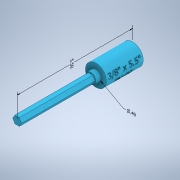
# Autodesk Inventor part: 3_8x7_5-inchHexShaft
Saved by Autodesk Inventor 2022.2 (Build 262287030, 287C)
## iProperties
Created: 2020-11-17
Part Number: 3_8x7_5-inchHexShaft
Material: PC/ABS Plastic
Document SubType Name: Modeling
Designer: robst
Density: 0.357273 g/cm^3
Appearance: Turquoise
Author: robst
Autodesk Inventor part; units mm, degrees
ref_plane "XZ Plane" through (0, 0, 0) normal (0, 1, 0) x (-1, 0, 0)
ref_plane "XY Plane" through (0, 0, 0) normal (0, 0, 1) x (1, 0, 0)
sketch "Sketch1" plane through (0, 0, 0) normal (0, 0, 1) x (1, 0, 0)
  line L0 (5.4993, 0) -> (2.7496, -4.7625)
  line L1 (2.7496, -4.7625) -> (-2.7496, -4.7625)
  line L2 (-2.7496, -4.7625) -> (-5.4993, 0)
  line L3 (-5.4993, 0) -> (-2.7496, 4.7625)
  line L4 (-2.7496, 4.7625) -> (2.7496, 4.7625)
  line L5 (2.7496, 4.7625) -> (5.4993, 0)
  circle A0 centre (0, 0) radius 0.0127
  dimension "d0" = 9.525
  dimension "d6" = 0.0254
  constraints: 12 end point, 2 coincident, 1 centre point, 1 horizontal, 13 other
  measures "d0" distance between parallel lines of L1 L4
  measures "d6" diameter of A0
extrude "Extrusion2" add sketch "Sketch1" along normal mid plane 114.3
sketch "Sketch4" plane through (0, 0, -57.15) normal (0, 0, -1) x (-1, 0, 0)
  circle A0 centre (0, 0) radius 0.0127 projected
  circle A1 centre (0, 0) radius 12.7
  dimension "d10" = 25.4
  constraints: 1 centre point, 1 coincident
  measures "d10" diameter of A1
extrude "Extrusion4" add sketch "Sketch4" against normal blind 19.05
thicken "Reduce Hex Shaft" operation add thickness 0.127 both sides no extend neighbours yes toward (0, -1, 0) faces at (0.9165, 4.7625, -6.35) (4.5827, 1.5875, -6.35) (3.6662, -3.175, -6.35) (-3.6662, 3.175, -6.35) (-4.5827, -1.5875, -6.35) (-0.9165, -4.7625, -6.35)
sketch "Sketch5" plane through (0, 0, -38.1) normal (0, 0, 1) x (1, 0, 0)
  circle A0 centre (0, 0) radius 6.35
  dimension "d15" = 12.7
  constraints: 1 centre point, 1 coincident
  measures "d15" diameter of A0
extrude "Extrusion5" add sketch "Sketch5" along normal blind 6.35
thicken "Reduce Base Bushing" operation add thickness 0.127 both sides no extend neighbours yes toward (-0.9967573, 0.0804666, 0) faces at (6.3294, -0.511, -33.8667)
sketch "Sketch8" plane through (0, 0, -57.15) normal (0, 0, -1) x (-1, 0, 0)
  circle A0 centre (0, 0) radius 12.7
  circle A1 centre (0, 0) radius 12.7 projected
  constraints: 1 centre point, 1 coincident, 1 concentric
extrude "Extrusion7" add sketch "Sketch8" along normal blind 25.4
ref_plane "Work Plane1" through (12.7, 0, -57.15) normal (1, 0, 0) x (0, 1, 0)
sketch "Sketch10" plane through (12.7, 0, -57.15) normal (1, 0, 0) x (0, 1, 0)
  line L0 (-12.7, -25.4) -> (12.7, -25.4) projected
  line L1 (12.7, 19.05) -> (-12.7, 19.05) projected
  line L2 (-6.223, 19.05) -> (6.223, 19.05) construction
  line L3 (0, 19.05) -> (0, -25.4) construction
  spline S0 degree 2 poles (5.518, 14.8141) (5.518, 15.0364) (5.4093, 15.4761) (5.3254, 15.6885) knots 0 0 0 1 2 2 2
  spline S1 degree 2 poles (5.3254, 15.6885) (5.2414, 15.8861) (5.0635, 16.1776) (4.9845, 16.2912) knots 0 0 0 1 2 2 2
  line L4 (4.9845, 16.2912) -> (4.9845, 16.3406)
  line L5 (4.9845, 16.3406) -> (5.849, 16.3406)
  spline S2 degree 2 poles (5.849, 16.3406) (5.9923, 16.0738) (6.2244, 15.1599) (6.2244, 14.7499) knots 0 0 0 1 2 2 2
  spline S3 degree 2 poles (6.2244, 14.7499) (6.2244, 14.3349) (6.0565, 13.7174) (5.8786, 13.4655) knots 0 0 0 1 2 2 2
  spline S4 degree 2 poles (5.8786, 13.4655) (5.686, 13.1987) (5.1278, 12.9221) (4.7523, 12.9221) knots 0 0 0 1 2 2 2
  spline S5 degree 2 poles (4.7523, 12.9221) (4.2484, 12.9221) (3.4877, 13.5841) (3.3889, 14.0484) knots 0 0 0 1 2 2 2
  line L6 (3.3889, 14.0484) -> (3.3296, 14.0484)
  spline S6 degree 2 poles (3.3296, 14.0484) (3.2901, 13.8558) (3.1122, 13.4161) (2.9344, 13.2284) knots 0 0 0 1 2 2 2
  spline S7 degree 2 poles (2.9344, 13.2284) (2.7615, 13.0407) (2.2082, 12.8035) (1.8081, 12.8035) knots 0 0 0 1 2 2 2
  spline S8 degree 2 poles (1.8081, 12.8035) (1.398, 12.8035) (0.7015, 13.0851) (0.4347, 13.342) knots 0 0 0 1 2 2 2
  spline S9 degree 2 poles (0.4347, 13.342) (0.1581, 13.6088) (-0.1284, 14.3646) (-0.1284, 14.8438) knots 0 0 0 1 2 2 2
  spline S10 degree 2 poles (-0.1284, 14.8438) (-0.1284, 15.3032) (0.0939, 16.2023) (0.247, 16.5086) knots 0 0 0 1 2 2 2
  line L7 (0.247, 16.5086) -> (1.1115, 16.5086)
  line L8 (1.1115, 16.5086) -> (1.1115, 16.4493)
  spline S11 degree 2 poles (1.1115, 16.4493) (0.9238, 16.1924) (0.578, 15.323) (0.578, 14.8932) knots 0 0 0 1 2 2 2
  spline S12 degree 2 poles (0.578, 14.8932) (0.578, 14.6412) (0.7361, 14.1373) (0.9188, 13.9694) knots 0 0 0 1 2 2 2
  spline S13 degree 2 poles (0.9188, 13.9694) (1.1016, 13.8064) (1.5364, 13.6335) (1.8673, 13.6335) knots 0 0 0 1 2 2 2
  spline S14 degree 2 poles (1.8673, 13.6335) (2.1983, 13.6335) (2.6281, 13.8261) (2.7516, 13.999) knots 0 0 0 1 2 2 2
  spline S15 degree 2 poles (2.7516, 13.999) (2.8751, 14.1719) (2.969, 14.6412) (2.969, 14.9179) knots 0 0 0 1 2 2 2
  line L9 (2.969, 14.9179) -> (2.969, 15.2637)
  line L10 (2.969, 15.2637) -> (3.6457, 15.2637)
  line L11 (3.6457, 15.2637) -> (3.6457, 14.992)
  spline S16 degree 2 poles (3.6457, 14.992) (3.6457, 14.4436) (4.1694, 13.752) (4.6683, 13.752) knots 0 0 0 1 2 2 2
  spline S17 degree 2 poles (4.6683, 13.752) (4.9005, 13.752) (5.2315, 13.9299) (5.3303, 14.0731) knots 0 0 0 1 2 2 2
  spline S18 degree 2 poles (5.3303, 14.0731) (5.434, 14.2263) (5.518, 14.6017) (5.518, 14.8141) knots 0 0 0 1 2 2 2
  line L12 (6.3677, 9.3505) -> (-1.3239, 11.7365)
  line L13 (-1.3239, 11.7365) -> (-1.3239, 12.4281)
  line L14 (-1.3239, 12.4281) -> (6.3677, 10.0519)
  line L15 (6.3677, 10.0519) -> (6.3677, 9.3505)
  spline S19 degree 2 poles (-0.1383, 6.836) (-0.1383, 7.2905) (0.1334, 8.0364) (0.3853, 8.2982) knots 0 0 0 1 2 2 2
  spline S20 degree 2 poles (0.3853, 8.2982) (0.6323, 8.5551) (1.3042, 8.8219) (1.6846, 8.8219) knots 0 0 0 1 2 2 2
  spline S21 degree 2 poles (1.6846, 8.8219) (2.1786, 8.8219) (3.0085, 8.2933) (3.2555, 7.7894) knots 0 0 0 1 2 2 2
  line L16 (3.2555, 7.7894) -> (3.2802, 7.7894)
  spline S22 degree 2 poles (3.2802, 7.7894) (3.542, 8.2389) (4.1644, 8.6737) (4.6288, 8.6737) knots 0 0 0 1 2 2 2
  spline S23 degree 2 poles (4.6288, 8.6737) (5.3155, 8.6737) (6.2343, 7.6363) (6.2343, 6.836) knots 0 0 0 1 2 2 2
  spline S24 degree 2 poles (6.2343, 6.836) (6.2343, 6.0061) (5.3649, 5.0032) (4.6832, 5.0032) knots 0 0 0 1 2 2 2
  spline S25 degree 2 poles (4.6832, 5.0032) (4.2731, 5.0032) (3.4728, 5.4824) (3.2456, 5.9319) knots 0 0 0 1 2 2 2
  line L17 (3.2456, 5.9319) -> (3.2209, 5.9319)
  spline S26 degree 2 poles (3.2209, 5.9319) (2.9739, 5.3984) (2.2625, 4.8501) (1.6994, 4.8501) knots 0 0 0 1 2 2 2
  spline S27 degree 2 poles (1.6994, 4.8501) (0.9188, 4.8501) (-0.1383, 5.9863) (-0.1383, 6.836) knots 0 0 0 1 2 2 2
  spline S28 degree 2 poles (1.6203, 5.6899) (1.9958, 5.6899) (2.4404, 5.9863) (2.6676, 6.4062) knots 0 0 0 1 2 2 2
  spline S29 degree 2 poles (2.6676, 6.4062) (2.7467, 6.5445) (2.9294, 7.0089) (3.048, 7.3003) knots 0 0 0 1 2 2 2
  spline S30 degree 2 poles (3.048, 7.3003) (2.8257, 7.6363) (2.1637, 7.9969) (1.7438, 7.9969) knots 0 0 0 1 2 2 2
  spline S31 degree 2 poles (1.7438, 7.9969) (1.1905, 7.9969) (0.4693, 7.33) (0.4693, 6.8261) knots 0 0 0 1 2 2 2
  spline S32 degree 2 poles (0.4693, 6.8261) (0.4693, 6.3123) (1.0868, 5.6899) (1.6203, 5.6899) knots 0 0 0 1 2 2 2
  spline S33 degree 2 poles (4.6733, 5.8035) (5.0833, 5.8035) (5.6316, 6.3519) (5.6316, 6.8409) knots 0 0 0 1 2 2 2
  spline S34 degree 2 poles (5.6316, 6.8409) (5.6316, 7.2855) (5.1426, 7.8536) (4.7227, 7.8536) knots 0 0 0 1 2 2 2
  spline S35 degree 2 poles (4.7227, 7.8536) (4.4213, 7.8536) (4.0014, 7.5622) (3.8335, 7.2707) knots 0 0 0 1 2 2 2
  spline S36 degree 2 poles (3.8335, 7.2707) (3.7643, 7.1472) (3.5222, 6.6236) (3.4531, 6.4111) knots 0 0 0 1 2 2 2
  spline S37 degree 2 poles (3.4531, 6.4111) (3.7248, 6.0555) (4.3028, 5.8035) (4.6733, 5.8035) knots 0 0 0 1 2 2 2
  line L18 (6.3677, 1.6489) -> (3.9965, 1.8268)
  line L19 (3.9965, 1.8268) -> (3.9965, 2.3652)
  line L20 (3.9965, 2.3652) -> (6.3677, 2.5431)
  line L21 (6.3677, 2.5431) -> (6.3677, 1.6489)
  line L22 (6.3677, 3.1902) -> (3.9965, 3.3681)
  line L23 (3.9965, 3.3681) -> (3.9965, 3.9065)
  line L24 (3.9965, 3.9065) -> (6.3677, 4.0844)
  line L25 (6.3677, 4.0844) -> (6.3677, 3.1902)
  line L26 (0, -5.5437) -> (0, -4.6002)
  line L27 (0, -4.6002) -> (1.7191, -3.4887)
  line L28 (1.7191, -3.4887) -> (0, -2.3475)
  line L29 (0, -2.3475) -> (0, -1.4732)
  line L30 (0, -1.4732) -> (2.2675, -3.0589)
  line L31 (2.2675, -3.0589) -> (4.5745, -1.488)
  line L32 (4.5745, -1.488) -> (4.5745, -2.4315)
  line L33 (4.5745, -2.4315) -> (2.8702, -3.5381)
  line L34 (2.8702, -3.5381) -> (4.5745, -4.6694)
  line L35 (4.5745, -4.6694) -> (4.5745, -5.5437)
  line L36 (4.5745, -5.5437) -> (2.3169, -3.9679)
  line L37 (2.3169, -3.9679) -> (0, -5.5437)
  spline S38 degree 2 poles (1.9365, -12.3412) (1.4968, -12.3412) (0.7459, -12.0596) (0.4693, -11.8028) knots 0 0 0 1 2 2 2
  spline S39 degree 2 poles (0.4693, -11.8028) (0.1927, -11.5459) (-0.1284, -10.7802) (-0.1284, -10.3059) knots 0 0 0 1 2 2 2
  spline S40 degree 2 poles (-0.1284, -10.3059) (-0.1284, -9.8712) (0.0642, -9.0215) (0.2174, -8.7103) knots 0 0 0 1 2 2 2
  line L38 (0.2174, -8.7103) -> (1.0819, -8.7103)
  line L39 (1.0819, -8.7103) -> (1.0819, -8.7696)
  spline S41 degree 2 poles (1.0819, -8.7696) (1.0127, -8.8634) (0.8349, -9.2142) (0.7558, -9.4266) knots 0 0 0 1 2 2 2
  spline S42 degree 2 poles (0.7558, -9.4266) (0.6718, -9.6687) (0.578, -10.0688) (0.578, -10.3208) knots 0 0 0 1 2 2 2
  spline S43 degree 2 poles (0.578, -10.3208) (0.578, -10.5678) (0.7558, -11.0321) (0.9485, -11.2001) knots 0 0 0 1 2 2 2
  spline S44 degree 2 poles (0.9485, -11.2001) (1.1313, -11.3532) (1.6154, -11.5113) (1.9414, -11.5113) knots 0 0 0 1 2 2 2
  spline S45 degree 2 poles (1.9414, -11.5113) (2.2675, -11.5113) (2.6824, -11.3335) (2.8208, -11.1655) knots 0 0 0 1 2 2 2
  spline S46 degree 2 poles (2.8208, -11.1655) (2.9739, -10.9926) (3.1023, -10.4788) (3.1023, -10.1676) knots 0 0 0 1 2 2 2
  spline S47 degree 2 poles (3.1023, -10.1676) (3.1023, -9.8317) (2.9986, -9.1648) (2.9541, -8.9622) knots 0 0 0 1 2 2 2
  line L40 (2.9541, -8.9622) -> (6.096, -8.9622)
  line L41 (6.096, -8.9622) -> (6.096, -12.3066)
  line L42 (6.096, -12.3066) -> (5.3797, -12.3066)
  line L43 (5.3797, -12.3066) -> (5.3797, -9.7477)
  line L44 (5.3797, -9.7477) -> (3.7544, -9.7477)
  spline S48 degree 2 poles (3.7544, -9.7477) (3.7742, -9.8959) (3.789, -10.1824) (3.789, -10.301) knots 0 0 0 1 2 2 2
  spline S49 degree 2 poles (3.789, -10.301) (3.789, -10.7703) (3.6359, -11.4174) (3.4086, -11.7138) knots 0 0 0 1 2 2 2
  spline S50 degree 2 poles (3.4086, -11.7138) (3.1814, -12.0152) (2.4898, -12.3412) (1.9365, -12.3412) knots 0 0 0 1 2 2 2
  line L45 (0, -14.5297) -> (0, -13.5515)
  line L46 (0, -13.5515) -> (1.1658, -13.5515)
  line L47 (1.1658, -13.5515) -> (1.1658, -14.5297)
  line L48 (1.1658, -14.5297) -> (0, -14.5297)
  spline S51 degree 2 poles (1.9365, -19.4549) (1.4968, -19.4549) (0.7459, -19.1733) (0.4693, -18.9164) knots 0 0 0 1 2 2 2
  spline S52 degree 2 poles (0.4693, -18.9164) (0.1927, -18.6595) (-0.1284, -17.8938) (-0.1284, -17.4196) knots 0 0 0 1 2 2 2
  spline S53 degree 2 poles (-0.1284, -17.4196) (-0.1284, -16.9849) (0.0642, -16.1352) (0.2174, -15.824) knots 0 0 0 1 2 2 2
  line L49 (0.2174, -15.824) -> (1.0819, -15.824)
  line L50 (1.0819, -15.824) -> (1.0819, -15.8832)
  spline S54 degree 2 poles (1.0819, -15.8832) (1.0127, -15.9771) (0.8349, -16.3278) (0.7558, -16.5403) knots 0 0 0 1 2 2 2
  spline S55 degree 2 poles (0.7558, -16.5403) (0.6718, -16.7823) (0.578, -17.1825) (0.578, -17.4344) knots 0 0 0 1 2 2 2
  spline S56 degree 2 poles (0.578, -17.4344) (0.578, -17.6814) (0.7558, -18.1458) (0.9485, -18.3137) knots 0 0 0 1 2 2 2
  spline S57 degree 2 poles (0.9485, -18.3137) (1.1313, -18.4669) (1.6154, -18.625) (1.9414, -18.625) knots 0 0 0 1 2 2 2
  spline S58 degree 2 poles (1.9414, -18.625) (2.2675, -18.625) (2.6824, -18.4471) (2.8208, -18.2791) knots 0 0 0 1 2 2 2
  spline S59 degree 2 poles (2.8208, -18.2791) (2.9739, -18.1062) (3.1023, -17.5925) (3.1023, -17.2813) knots 0 0 0 1 2 2 2
  spline S60 degree 2 poles (3.1023, -17.2813) (3.1023, -16.9453) (2.9986, -16.2784) (2.9541, -16.0759) knots 0 0 0 1 2 2 2
  line L51 (2.9541, -16.0759) -> (6.096, -16.0759)
  line L52 (6.096, -16.0759) -> (6.096, -19.4203)
  line L53 (6.096, -19.4203) -> (5.3797, -19.4203)
  line L54 (5.3797, -19.4203) -> (5.3797, -16.8614)
  line L55 (5.3797, -16.8614) -> (3.7544, -16.8614)
  spline S61 degree 2 poles (3.7544, -16.8614) (3.7742, -17.0096) (3.789, -17.2961) (3.789, -17.4146) knots 0 0 0 1 2 2 2
  spline S62 degree 2 poles (3.789, -17.4146) (3.789, -17.8839) (3.6359, -18.5311) (3.4086, -18.8275) knots 0 0 0 1 2 2 2
  spline S63 degree 2 poles (3.4086, -18.8275) (3.1814, -19.1288) (2.4898, -19.4549) (1.9365, -19.4549) knots 0 0 0 1 2 2 2
  line L56 (6.3677, -21.2481) -> (3.9965, -21.0703)
  line L57 (3.9965, -21.0703) -> (3.9965, -20.5318)
  line L58 (3.9965, -20.5318) -> (6.3677, -20.354)
  line L59 (6.3677, -20.354) -> (6.3677, -21.2481)
  line L60 (6.3677, -22.7894) -> (3.9965, -22.6116)
  line L61 (3.9965, -22.6116) -> (3.9965, -22.0731)
  line L62 (3.9965, -22.0731) -> (6.3677, -21.8953)
  line L63 (6.3677, -21.8953) -> (6.3677, -22.7894)
  spline S64 degree 2 poles (-5.8084, 3.2643) (-6.2036, 3.2643) (-6.9149, 3.5459) (-7.1619, 3.7979) knots 0 0 0 1 2 2 2
  spline S65 degree 2 poles (-7.1619, 3.7979) (-7.4732, 4.114) (-7.7943, 4.9686) (-7.7943, 5.6207) knots 0 0 0 1 2 2 2
  line L64 (-7.7943, 5.6207) -> (-7.7943, 6.3074)
  line L65 (-7.7943, 6.3074) -> (-10.0667, 6.3074)
  line L66 (-10.0667, 6.3074) -> (-10.0667, 7.1176)
  line L67 (-10.0667, 7.1176) -> (-3.9707, 7.1176)
  line L68 (-3.9707, 7.1176) -> (-3.9707, 5.5861)
  spline S66 degree 2 poles (-3.9707, 5.5861) (-3.9707, 5.0427) (-4.1485, 4.282) (-4.3511, 3.9905) knots 0 0 0 1 2 2 2
  spline S67 degree 2 poles (-4.3511, 3.9905) (-4.5832, 3.6497) (-5.2996, 3.2643) (-5.8084, 3.2643) knots 0 0 0 1 2 2 2
  spline S68 degree 2 poles (-5.8331, 4.1091) (-5.5169, 4.1091) (-5.0526, 4.3264) (-4.9044, 4.5487) knots 0 0 0 1 2 2 2
  spline S69 degree 2 poles (-4.9044, 4.5487) (-4.7759, 4.7414) (-4.6722, 5.2552) (-4.6722, 5.6355) knots 0 0 0 1 2 2 2
  line L69 (-4.6722, 5.6355) -> (-4.6722, 6.3074)
  line L70 (-4.6722, 6.3074) -> (-7.1027, 6.3074)
  line L71 (-7.1027, 6.3074) -> (-7.1027, 5.7541)
  spline S70 degree 2 poles (-7.1027, 5.7541) (-7.1027, 5.2601) (-6.9446, 4.6525) (-6.7371, 4.4549) knots 0 0 0 1 2 2 2
  spline S71 degree 2 poles (-6.7371, 4.4549) (-6.5543, 4.2721) (-6.1245, 4.1091) (-5.8331, 4.1091) knots 0 0 0 1 2 2 2
  line L72 (-3.9707, -1.9276) -> (-10.0667, 0.1719)
  line L73 (-10.0667, 0.1719) -> (-10.0667, 1.0463)
  line L74 (-10.0667, 1.0463) -> (-3.9707, 3.1458)
  line L75 (-3.9707, 3.1458) -> (-3.9707, 2.2763)
  line L76 (-3.9707, 2.2763) -> (-9.0342, 0.5868)
  line L77 (-9.0342, 0.5868) -> (-3.9707, -1.1027)
  line L78 (-3.9707, -1.1027) -> (-3.9707, -1.9276)
  line L79 (-7.7696, -4.6397) -> (-7.7696, -2.3327)
  line L80 (-7.7696, -2.3327) -> (-7.0286, -2.3327)
  line L81 (-7.0286, -2.3327) -> (-7.0286, -4.6397)
  line L82 (-7.0286, -4.6397) -> (-7.7696, -4.6397)
  spline S72 degree 2 poles (-7.0187, -9.2438) (-8.6588, -9.2438) (-10.1951, -8.2904) (-10.1951, -7.2975) knots 0 0 0 1 2 2 2
  spline S73 degree 2 poles (-10.1951, -7.2975) (-10.1951, -6.2897) (-8.6291, -5.3461) (-7.0236, -5.3461) knots 0 0 0 1 2 2 2
  spline S74 degree 2 poles (-7.0236, -5.3461) (-5.3737, -5.3461) (-3.8472, -6.2996) (-3.8472, -7.2975) knots 0 0 0 1 2 2 2
  spline S75 degree 2 poles (-3.8472, -7.2975) (-3.8472, -8.3003) (-5.428, -9.2438) (-7.0187, -9.2438) knots 0 0 0 1 2 2 2
  spline S76 degree 2 poles (-8.8761, -8.1965) (-8.5748, -8.3151) (-7.6461, -8.4139) (-7.0187, -8.4139) knots 0 0 0 1 2 2 2
  spline S77 degree 2 poles (-7.0187, -8.4139) (-6.3913, -8.4139) (-5.4675, -8.3151) (-5.1563, -8.1916) knots 0 0 0 1 2 2 2
  spline S78 degree 2 poles (-5.1563, -8.1916) (-4.8451, -8.0681) (-4.524, -7.6383) (-4.524, -7.2975) knots 0 0 0 1 2 2 2
  spline S79 degree 2 poles (-4.524, -7.2975) (-4.524, -6.9566) (-4.8451, -6.5169) (-5.1662, -6.3885) knots 0 0 0 1 2 2 2
  spline S80 degree 2 poles (-5.1662, -6.3885) (-5.4774, -6.265) (-6.4259, -6.1761) (-7.0236, -6.1761) knots 0 0 0 1 2 2 2
  spline S81 degree 2 poles (-7.0236, -6.1761) (-7.6658, -6.1761) (-8.5254, -6.2551) (-8.8613, -6.3836) knots 0 0 0 1 2 2 2
  spline S82 degree 2 poles (-8.8613, -6.3836) (-9.1775, -6.5021) (-9.5183, -6.9418) (-9.5183, -7.2975) knots 0 0 0 1 2 2 2
  spline S83 degree 2 poles (-9.5183, -7.2975) (-9.5183, -7.6334) (-9.1972, -8.073) (-8.8761, -8.1965) knots 0 0 0 1 2 2 2
  line L83 (-10.0667, -13.7837) -> (-10.0667, -10.0244)
  line L84 (-10.0667, -10.0244) -> (-9.2022, -10.0244)
  spline S84 degree 2 poles (-9.2022, -10.0244) (-8.8218, -10.4294) (-8.1154, -11.1507) (-7.735, -11.4965) knots 0 0 0 1 2 2 2
  spline S85 degree 2 poles (-7.735, -11.4965) (-6.9693, -12.193) (-6.0504, -12.7019) (-5.5614, -12.7019) knots 0 0 0 1 2 2 2
  spline S86 degree 2 poles (-5.5614, -12.7019) (-5.3045, -12.7019) (-4.9192, -12.5438) (-4.7957, -12.4005) knots 0 0 0 1 2 2 2
  spline S87 degree 2 poles (-4.7957, -12.4005) (-4.6722, -12.2572) (-4.5487, -11.8818) (-4.5487, -11.6546) knots 0 0 0 1 2 2 2
  spline S88 degree 2 poles (-4.5487, -11.6546) (-4.5487, -11.4372) (-4.6574, -10.9926) (-4.7413, -10.7901) knots 0 0 0 1 2 2 2
  spline S89 degree 2 poles (-4.7413, -10.7901) (-4.8105, -10.6172) (-5.0081, -10.2961) (-5.0773, -10.1973) knots 0 0 0 1 2 2 2
  line L85 (-5.0773, -10.1973) -> (-5.0773, -10.1528)
  line L86 (-5.0773, -10.1528) -> (-4.2078, -10.1528)
  spline S90 degree 2 poles (-4.2078, -10.1528) (-4.0843, -10.4047) (-3.8422, -11.3088) (-3.8422, -11.7138) knots 0 0 0 1 2 2 2
  spline S91 degree 2 poles (-3.8422, -11.7138) (-3.8422, -12.5685) (-4.7463, -13.5318) (-5.5169, -13.5318) knots 0 0 0 1 2 2 2
  spline S92 degree 2 poles (-5.5169, -13.5318) (-5.8775, -13.5318) (-6.4802, -13.3638) (-6.7371, -13.2156) knots 0 0 0 1 2 2 2
  spline S93 degree 2 poles (-6.7371, -13.2156) (-7.0039, -13.0674) (-7.5275, -12.6376) (-7.7795, -12.4005) knots 0 0 0 1 2 2 2
  spline S94 degree 2 poles (-7.7795, -12.4005) (-8.1994, -12.0152) (-9.0984, -11.0716) (-9.3603, -10.7901) knots 0 0 0 1 2 2 2
  line L87 (-9.3603, -10.7901) -> (-9.3603, -13.7837)
  line L88 (-9.3603, -13.7837) -> (-10.0667, -13.7837)
  point P0 (0, 57.15)
  constraints: 2 end point, 2 midpoint, 1 vertical
emboss "Emboss3" sketch "Sketch10" operation cut depth 2.54 direction (-1, 0, 0) wrap yes faces at (-12.5355, -2.0372, -52.9167)
sketch "Sketch11" plane through (0, 0, -82.55) normal (0, 0, -1) x (-1, 0, 0)
  line L0 (3.8128, 6.604) -> (7.6256, 0)
  line L1 (7.6256, 0) -> (3.8128, -6.604)
  line L2 (3.8128, -6.604) -> (-3.8128, -6.604)
  line L3 (-3.8128, -6.604) -> (-7.6256, 0)
  line L4 (-7.6256, 0) -> (-3.8128, 6.604)
  line L5 (-3.8128, 6.604) -> (3.8128, 6.604)
  point P0 (0, 0)
  point P1 (0, 0)
  dimension "d39" = 13.208
  constraints: 12 end point, 1 coincident, 1 horizontal, 13 other
  measures "d39" distance between parallel lines of L2 L5
extrude "Extrusion8" cut sketch "Sketch11" against normal blind 38.1
equation "\"d0\" = hexSize"
equation "\"d4\" = length"
equation "\"d13\" = printOffset"
equation "\"d14\" = printOffset"
equation "\"d15\" = bushingForBaseHole"
equation "\"d16\" = sideOfBase"
equation "\"d20\" = printOffset"
equation "\"d21\" = printOffset"
equation "\"hexSize\" = 9.525"
equation "\"length\" = 114.3"
equation "\"printOffset\" = 0.127"
equation "\"bushingForBaseHole\" = 12.7"
equation "\"sideOfBase\" = 6.35"
body "Solid2"
